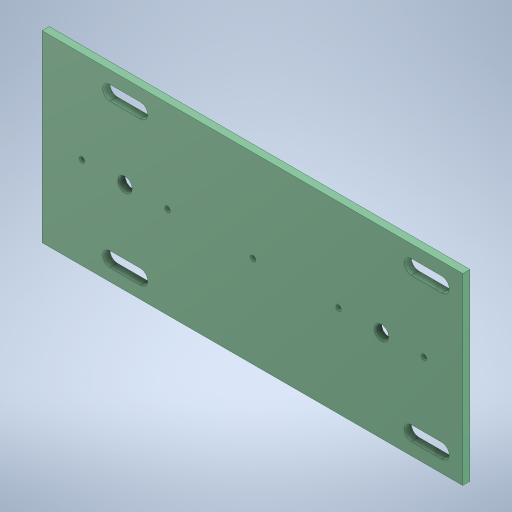
# Autodesk Inventor part: PCB SiPM 4CH corta
Saved by Autodesk Inventor 2024.2 (Build 282272000, 272)
## iProperties
Created: 2024-08-30
Part Number: PCB SiPM 4CH corta
Material: Phenolic Resin
Document SubType Name: Modeling
Designer: ja.restrepo1
Density: 1.38 g/cm^3
Appearance: Smooth - Dark Sea Green
Author: ja.restrepo1
Autodesk Inventor part; units mm, degrees
ref_plane "YZ Plane" through (0, 0, 0) normal (1, 0, 0) x (0, 1, 0)
ref_plane "XZ Plane" through (0, 0, 0) normal (0, 1, 0) x (-1, 0, 0)
ref_plane "XY Plane" through (0, 0, 0) normal (0, 0, 1) x (1, 0, 0)
sketch "Sketch1" plane through (0, 0, 0) normal (0, 0, 1) x (1, 0, 0)
  line L0 (-46.75, 20.4) -> (46.75, 20.4)
  line L1 (46.75, 20.4) -> (46.75, -20.4)
  line L2 (46.75, -20.4) -> (-46.75, -20.4)
  line L3 (-46.75, -20.4) -> (-46.75, 20.4)
  line L4 (-31.65, 16) -> (-24.85, 16) construction
  line L5 (-31.65, 14.4) -> (-24.85, 14.4)
  line L6 (-24.85, 17.6) -> (-31.65, 17.6)
  arc A0 (-31.65, 17.6) -> (-31.65, 14.4) centre (-31.65, 16) ccw
  arc A1 (-24.85, 14.4) -> (-24.85, 17.6) centre (-24.85, 16) ccw
  line L7 (-31.65, -16) -> (-24.85, -16) construction
  line L8 (-31.65, -17.6) -> (-24.85, -17.6)
  line L9 (-24.85, -14.4) -> (-31.65, -14.4)
  arc A2 (-31.65, -14.4) -> (-31.65, -17.6) centre (-31.65, -16) ccw
  arc A3 (-24.85, -17.6) -> (-24.85, -14.4) centre (-24.85, -16) ccw
  line L10 (35.35, 16) -> (42.15, 16) construction
  line L11 (35.35, 14.4) -> (42.15, 14.4)
  line L12 (42.15, 17.6) -> (35.35, 17.6)
  arc A4 (35.35, 17.6) -> (35.35, 14.4) centre (35.35, 16) ccw
  arc A5 (42.15, 14.4) -> (42.15, 17.6) centre (42.15, 16) ccw
  line L13 (35.35, -16) -> (42.15, -16) construction
  line L14 (35.35, -17.6) -> (42.15, -17.6)
  line L15 (42.15, -14.4) -> (35.35, -14.4)
  arc A6 (35.35, -14.4) -> (35.35, -17.6) centre (35.35, -16) ccw
  arc A7 (42.15, -17.6) -> (42.15, -14.4) centre (42.15, -16) ccw
  line L16 (-28.25, 16) -> (-28.25, -16) construction
  line L17 (-28.25, -16) -> (38.75, -16) construction
  circle A8 centre (28.7, 0) radius 1.6
  circle A9 centre (-28.3, 0) radius 1.6
  circle A10 centre (38.15, 0) radius 0.6
  circle A11 centre (19.15, 0) radius 0.6
  circle A12 centre (0.15, 0) radius 0.6
  circle A13 centre (-18.85, 0) radius 0.6
  circle A14 centre (-37.85, 0) radius 0.6
  point P0 (0, 0)
  point P1 (0, 20.4)
  point P2 (-46.75, 0)
  point P3 (38.75, 16)
  point P4 (-28.25, 0)
  dimension "d0" = 40.8
  dimension "d1" = 93.5
  dimension "d2" = 3.2
  dimension "d3" = 3.2
  dimension "d4" = 3.2
  dimension "d5" = 3.2
  dimension "d6" = 32
  dimension "d7" = 67
  dimension "d8" = 4.6
  dimension "d9" = 6.8
  dimension "d10" = 3.2
  dimension "d11" = 57
  dimension "d13" = 1.2
  dimension "d14" = 8.6
  dimension "d15" = 1.2
  dimension "d16" = 1.2
  dimension "d17" = 1.2
  dimension "d18" = 1.2
  dimension "d20" = 19
  dimension "d21" = 19
  dimension "d22" = 19
  dimension "d23" = 19
  dimension "d27" = 18.05
  constraints: 44 end point, 16 point on circle, 16 tangent, 15 centre point, 11 horizontal alignment, 7 midpoint, 6 parallel, 5 horizontal, 3 equal length, 3 vertical alignment, 1 equal radius, 1 perpendicular
  measures "d0" distance of L2.end L0.start
  measures "d1" distance of L0.start L0.end
  measures "d2" diameter of A1
  measures "d3" diameter of A3
  measures "d4" diameter of A5
  measures "d5" diameter of A7
  measures "d6" distance of L16.start L16.end
  measures "d7" distance of L16.end L17.end
  measures "d8" distance from line of L13.end L1
  measures "d9" distance of L4.start L4.end
  measures "d10" diameter of A8
  measures "d11" distance of A9.centre A8.centre
  measures "d13" diameter of A10
  measures "d14" distance from line of A10.centre L1
  measures "d15" diameter of A11
  measures "d16" diameter of A12
  measures "d17" diameter of A13
  measures "d18" diameter of A14
  measures "d20" distance of A11.centre A10.centre
  measures "d21" distance of A12.centre A11.centre
  measures "d22" distance of A12.centre A13.centre
  measures "d23" distance of A14.centre A13.centre
  measures "d27" distance from line of L1 A8.centre
extrude "PCB SiPM 4CH corta" add sketch "Sketch1" along normal mid plane 1.6
equation "\"d21\" = d20"
equation "\"d22\" = d20"
equation "\"d23\" = d20"
body "Solid1"
